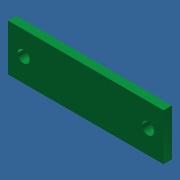
# Autodesk Inventor part: J002608
Saved by Autodesk Inventor 2012 SP2 (Build 160219200, 219)
## iProperties
Created: 2014-07-03
Material: Default
Vendor: HHMI: JFRC - ID&F
Document SubType Name: Modeling
Designer: NEGRASHOVI
Density: 1 g/cm^3
Part Number: J002608
RuleStatus: InUse
AfterDocSave0: file://Part Number Cleaner
DESIGN DEPARTMENT: HHMI: JFRC - ID&F
ALTERED ITEM PART NUMBER: N/A
ALTERED ITEM VENDOR: N/A
ALTERED ITEM DESCRIPTION: N/A
Author: NEGRASHOVI
Revision Number: 0
Autodesk Inventor part; units mm, degrees
ref_plane "YZ Plane" through (0, 0, 0) normal (1, 0, 0) x (0, 1, 0)
ref_plane "XZ Plane" through (0, 0, 0) normal (0, 1, 0) x (-1, 0, 0)
ref_plane "XY Plane" through (0, 0, 0) normal (0, 0, 1) x (1, 0, 0)
sketch "Sketch1" plane through (0, 0, 0) normal (0, 0, 1) x (1, 0, 0)
  line L0 (-15.875, -4.7625) -> (15.875, -4.7625)
  line L1 (15.875, -4.7625) -> (15.875, 4.7625)
  line L2 (15.875, 4.7625) -> (-15.875, 4.7625)
  line L3 (-15.875, 4.7625) -> (-15.875, -4.7625)
  line L4 (-15.875, -4.7625) -> (15.875, 4.7625) construction
  point P0 (0, 0)
  point P1 (0, 0)
  dimension "d0" = 31.75
  dimension "d1" = 9.525
  constraints: 10 end point, 2 parallel, 1 coincident, 1 horizontal, 1 midpoint, 1 perpendicular
  measures "d0" distance of L1.end L2.end
  measures "d1" distance of L2.end L0.start
extrude "Extrusion1" add sketch "Sketch1" along normal blind 1.7018
sketch "Sketch2" plane through (0, 0, 1.7018) normal (0, 0, 1) x (1, 0, 0)
  line L0 (-22.225, 0) -> (22.225, 0) construction
  line L1 (0, -6.6675) -> (0, 6.6675) construction
  circle A0 centre (-12.7, 0) radius 1.2192
  circle A1 centre (12.7, 0) radius 1.2192
  point P0 (0, 0)
  dimension "d4" = 25.4
  dimension "d5" = 2.4384
  constraints: 2 centre point, 2 point on line, 1 equal radius, 1 other
  measures "d4" distance of A1.centre A0.centre
  measures "d5" diameter of A0
extrude "Extrusion2" cut sketch "Sketch2" against normal through all
body "Solid1"
